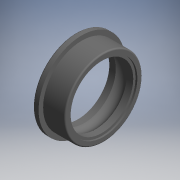
# Autodesk Inventor part: F606ZZ Outer Ring
Saved by Autodesk Inventor 2017.3 (Build 213256000, 256)
## iProperties
Part Number: F606ZZ Outer Ring
Material: Generic
Catalog Web Link: www.cadenas.de
Description: shielded_type_zz_zzs_OR-
Vendor: NSK_RB
Document SubType Name: Modeling
Designer: partserver
Manufacturer: NSK_RB
Mass: 0.47996 g
Surface Area: 8.63651 cm^2
Volume: 0.47996 cm^3
Density: 1 g/cm^3
Appearance: PSOLRGB-128-128-128
Category: PARTsolutions
Company: NSK_RB
Title: F606ZZ Outer Ring
Author: Cadenas PARTsolutions
PSOL_IDENT_0: {$CADENAS_DATA\23d-libs\nsk_rb\roller_bearings\deep_groove_bb\exstra_small_miniatur_bb\metric_design
PSOL_IDENT_1: _with_flange\shielded_type_zz_zzs_or1.prj},192 {VTYP=3D},{NB=F606ZZ Outer Ring},{LINA=F606ZZ Outer R
PSOL_IDENT_2: ing},{NN=shielded_type_zz_zzs_OR},{DATE=10.04.2020 04:57:39},{GEOMDATE=04.01.2008 00:00:00},{VERSION=
PSOL_IDENT_3: },{LINEID=540},{WBVAR=},{WBNUMERIC=}  {NB=F606ZZ Outer Ring},{LINA=F606ZZ Outer Ring},{KT=DUMMY},{ID
PSOL_IDENT_4: NR=},{STAN=},{ORDER=F606ZZ},{SD=6.0},{X=6.0},{D=17},{DD=17},{DD1=0.0},{D2=19.0},{DD2=19.0},{B=0.0},{
PSOL_IDENT_5: B1=6.0},{CC1=0.0},{C2=1.2},{CC2=1.2},{R=0.00},{R1=0.30},{DI1=8.92},{DI2=8.20},{SDE1=13.75},{SDE2=14.
PSOL_IDENT_6: 80},{CR1=2260},{COR1=835},{CR2=231},{COR2=85.0},{LG=38000},{LO=45000},{DA=0.0},{DB=8.2},{RA=0.00},{R
PSOL_IDENT_7: B=0.30},{MASS=6.61},{SC=1}
NB: F606ZZ Outer Ring
NN: shielded_type_zz_zzs_OR
NBSYN: $ORDER. Outer Ring
LINA: F606ZZ Outer Ring
CATALOG: NSK Rolling Bearing
ORDER: F606ZZ
SD: 6
X: 6
D: 17
DD: 17
DD1: 0
D2: 19
DD2: 19
B: 0
B1: 6
CC1: 0
C2: 1.2
CC2: 1.2
R: 0
R1: 0.3
DI1: 8.92
DI2: 8.2
SDE1: 13.75
SDE2: 14.8
CR1: 2260
COR1: 835
CR2: 231
COR2: 85
LG: 38000
LO: 45000
DA: 0
DB: 8.2
RA: 0
RB: 0.3
MASS: 6.61
SC: 1
SUPPLIER: NSK_RB
ARTICLENO: F606ZZ Outer Ring
BOMINFO: F606ZZ Outer Ring
CREATOR: CADENAS GmbH
Autodesk Inventor part; units mm, degrees
ref_plane "YZ Plane" through (0, 0, 0) normal (1, 0, 0) x (0, 1, 0)
ref_plane "XZ Plane" through (0, 0, 0) normal (0, 1, 0) x (-1, 0, 0)
ref_plane "XY Plane" through (0, 0, 0) normal (0, 0, 1) x (1, 0, 0)
sketch "Sketch_1" plane through (0, 0, 0) normal (0, 0, 1) x (1, 0, 0)
  line L0 (6, 0) -> (0, 0)
  line L1 (0, 7.4) -> (0.375, 7.4)
  line L2 (0.375, 7.4) -> (0.375, 6.875)
  line L3 (0.375, 6.875) -> (1.793, 6.875)
  arc A0 (4.207, 6.875) -> (1.793, 6.875) centre (3, 5.75) ccw
  line L4 (4.207, 6.875) -> (5.625, 6.875)
  line L5 (5.625, 6.875) -> (5.625, 7.4)
  line L6 (5.625, 7.4) -> (6, 7.4)
  line L7 (6, 7.4) -> (6, 9.2)
  arc A1 (6, 9.2) -> (5.7, 9.5) centre (5.7, 9.2) ccw
  line L8 (5.7, 9.5) -> (4.8, 9.5)
  line L9 (4.8, 9.5) -> (4.8, 8.5)
  line L10 (4.8, 8.5) -> (0.3, 8.5)
  arc A2 (0.3, 8.5) -> (0, 8.2) centre (0.3, 8.2) ccw
  line L11 (0, 8.2) -> (0, 7.4)
  constraints: 24 end point, 6 point on circle, 3 centre point
revolve "Revolution1" add sketch "Sketch_1" angle 360 about axis through (6, 0, 0) along (1, 0, 0)
ref_plane "ip_st_1_XY" through (0, 0, 0) normal (1, 0, 0) x (0, 0, -1)
ref_plane "ip_st_1_YZ" through (0, 0, 0) normal (0, 0, -1) x (0, 1, 0)
ref_plane "ip_st_1_ZX" through (0, 0, 0) normal (0, 1, 0) x (1, 0, 0)
ref_plane "ip_st_2_XY" through (5.625, 0, 0) normal (-1, 0, 0) x (0, 0, -1)
ref_plane "ip_st_2_YZ" through (5.625, 0, 0) normal (0, 0, -1) x (0, -1, 0)
ref_plane "ip_st_2_ZX" through (5.625, 0, 0) normal (0, -1, 0) x (-1, 0, 0)
body "Solid1"
